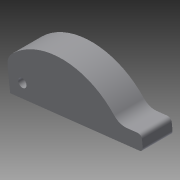
# Autodesk Inventor part: Surface Switch Trigger (Low Rider)
Saved by Autodesk Inventor 2015 (Build 190159000, 159)
## iProperties
Created: 2015-02-05
Part Number: Surface Switch Trigger (Low Rider)
Material: Generic
Document SubType Name: Modeling
Designer: robotics
Density: 1 g/cm^3
Appearance: Default
Author: robotics
Autodesk Inventor part; units mm, degrees
ref_plane "YZ Plane" through (0, 0, 0) normal (1, 0, 0) x (0, 1, 0)
ref_plane "XZ Plane" through (0, 0, 0) normal (0, 1, 0) x (-1, 0, 0)
ref_plane "XY Plane" through (0, 0, 0) normal (0, 0, 1) x (1, 0, 0)
sketch "Sketch1" plane through (0, 0, 0) normal (0, 0, 1) x (1, 0, 0)
  line L0 (-14.534, 1.5317) -> (13.0836, 4.6943)
  circle A0 centre (-11.9285, 4.7064) radius 0.889
  line L1 (10.3582, 7.5299) -> (12.7278, 7.8013)
  line L2 (13.7819, 5.5732) -> (13.6067, 7.103)
  arc A1 (13.6067, 7.103) -> (12.7278, 7.8013) centre (12.8181, 7.0127) ccw
  arc A2 (13.0836, 4.6943) -> (13.7819, 5.5732) centre (12.9933, 5.4829) ccw
  line L3 (32.8587, 7.8064) -> (-30.5519, 7.8064) construction
  line L4 (-30.2613, 13.1404) -> (33.8138, 13.1404) construction
  line L5 (-30.9672, 1.5317) -> (34.7689, 1.5317) construction
  line L6 (31.696, 4.6943) -> (-28.6002, 4.6943) construction
  line L7 (-29.3477, 13.3894) -> (32.568, 13.3894) construction
  line L8 (-30.5519, 10.5496) -> (32.8587, 10.5496) construction
  line L9 (17.7471, 10.5496) -> (27.535, 10.5496) construction
  line L10 (27.535, 10.5496) -> (27.535, 7.8064) construction
  line L11 (27.535, 7.8064) -> (17.7471, 7.8064) construction
  line L12 (17.7471, 7.8064) -> (17.7471, 10.5496) construction
  line L13 (17.7471, 13.1404) -> (27.535, 13.1404) construction
  line L14 (27.535, 13.1404) -> (27.535, 10.5496) construction
  line L15 (27.535, 10.5496) -> (17.7471, 10.5496) construction
  line L16 (17.7471, 10.5496) -> (17.7471, 13.1404) construction
  line L17 (-11.8273, 3.8231) -> (-11.6034, 1.8673) construction
  line L18 (-11.8273, 3.8231) -> (-11.8273, 1.5317) construction
  line L19 (-26.9329, 1.8545) -> (28.4398, 1.8545) construction
  line L20 (17.7471, 1.8545) -> (27.535, 1.8545) construction
  line L21 (27.535, 1.8545) -> (27.535, 1.5317) construction
  line L22 (27.535, 1.5317) -> (17.7471, 1.5317) construction
  line L23 (17.7471, 1.5317) -> (17.7471, 1.8545) construction
  line L24 (-15.1099, 1.5317) -> (-15.1099, 10.5496) construction
  line L25 (8.6645, 10.5496) -> (8.6645, 1.5317) construction
  line L26 (-14.534, 1.5317) -> (-15.0893, 6.3803)
  arc A3 (7.6693, 8.525) -> (-14.1664, 9) centre (-3.4787, -1.8171) ccw
  arc A4 (-14.1664, 9) -> (-15.0893, 6.3803) centre (-11.9349, 6.7415) ccw
  arc A5 (7.6693, 8.525) -> (10.3582, 7.5299) centre (9.997, 10.6843) ccw
  point P0 (8.6645, 7.336)
  point P1 (-15.2526, 7.8064)
  dimension "nail" = 1.778
  dimension "d38" = 0.7937
  dimension "d61" = 3.1273
  dimension "d62" = 27.7981
  dimension "d69" = 3.1625
  dimension "d71" = 2.7432
  dimension "d72" = 2.5908
  dimension "d73" = 1.9686
  dimension "d75" = 2.2914
  dimension "d76" = 0.3228
  dimension "d77" = 2.8397
  dimension "d78" = 23.7744
  dimension "d80" = 3.175
  constraints: 30 end point, 12 point on circle, 11 tangent, 10 collinear, 10 point on line, 7 horizontal, 7 perpendicular, 5 centre point, 3 parallel, 2 equal radius, 13 other
  measures "d38" radius of A1
  measures "d61" distance between parallel lines of L0 L1
  measures "d62" distance of L0.start L0.end
  measures "d69" distance between parallel lines of L5 L6
  measures "d71" distance between parallel lines of L3 L8
  measures "d72" distance between parallel lines of L8 L4
  measures "d73" distance of L17.start L17.end
  measures "d75" distance of L17.start L18.end
  measures "d76" distance between parallel lines of L5 L19
  measures "d77" distance between parallel lines of L8 L7
  measures "d78" distance between parallel lines of L25 L24
  measures "d80" radius of A4
extrude "Extrusion6" add sketch "Sketch1" along normal blind 6.35
body "Solid3"
